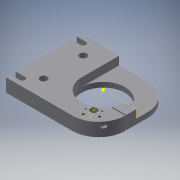
# Autodesk Inventor part: v2_tri_mount
Saved by Autodesk Inventor 2019 (Build 230136000, 136)
## iProperties
Created: 2017-03-10
Part Number: v2_tri_mount
Material: Generic
Document SubType Name: Modeling
Designer: richp
Density: 1 g/cm^3
Appearance: Default
mount_radius: 0.964 in
fov_diameter: 0.300 in
tri_angle: 120.00 deg
hole_diameter: 1.639 in
main_aperture_diameter: 1.639 in
Author: richp
Autodesk Inventor part; units mm, degrees
ref_plane "YZ Plane" through (0, 0, 0) normal (1, 0, 0) x (0, 1, 0)
ref_plane "XZ Plane" through (0, 0, 0) normal (0, 1, 0) x (-1, 0, 0)
ref_plane "XY Plane" through (0, 0, 0) normal (0, 0, 1) x (1, 0, 0)
sketch "Sketch1" plane through (0, 0, 0) normal (0, 1, 0) x (-1, 0, 0)
  line L0 (-54.2742, 0) -> (84.3226, 0) construction
  line L1 (-6.35, -36.068) -> (57.15, -36.068)
  line L2 (57.15, -36.068) -> (57.15, 36.068)
  line L3 (57.15, 36.068) -> (-6.35, 36.068)
  line L4 (-31.75, 10.668) -> (-31.75, -10.668)
  circle A0 centre (0, 0) radius 17 construction
  circle A1 centre (0, 0) radius 20.81
  line L5 (0, 0) -> (-18.9066, 32.7472) construction
  circle A2 centre (0, 0) radius 3.81 construction
  arc A3 (-6.35, 36.068) -> (-31.75, 10.668) centre (-6.35, 10.668) ccw
  arc A4 (-31.75, -10.668) -> (-6.35, -36.068) centre (-6.35, -10.668) ccw
  circle A5 centre (-12.2465, 21.2116) radius 1.6256 construction
  line L6 (0, 0) -> (31.1733, 53.9938) construction
  circle A6 centre (24.493, 0) radius 1.6256 construction
  circle A7 centre (-12.2465, -21.2116) radius 1.6256 construction
  circle A8 centre (-12.2465, 21.2116) radius 3.175 construction
  point P0 (-31.75, -36.068)
  point P1 (-31.75, 36.068)
  dimension "d0" = 72.136
  dimension "d1" = 88.9
  dimension "d2" = 34
  dimension "d3" = 3.81
  dimension "d4" = 31.75
  dimension "tri_angle" = 120
  dimension "fov_diameter" = 7.62
  dimension "d9" = 25.4
  dimension "d12" = 3.2512
  dimension "mount_radius" = 24.493
  dimension "d14" = 60
  dimension "d25" = 6.35
  dimension "main_aperture_diameter" = 41.62
  dimension "d67" = 2.0574
  dimension "d68" = 10.94
  constraints: 14 end point, 9 centre point, 6 point on line, 5 point on circle, 4 coincident, 4 tangent, 2 horizontal, 2 parallel, 2 symmetric about line, 1 equal radius, 1 perpendicular, 3 other
  measures "d0" distance of point (-31.75, 36.068) point (-31.75, -36.068)
  measures "d1" distance of L2.end point (-31.75, 36.068)
  measures "d2" diameter of A0
  measures "d3" radial gap between concentric circles of A1 A0
  measures "d4" distance from line of L5.start L4
  measures "tri_angle" angle of L0 L5
  measures "fov_diameter" diameter of A2
  measures "d9" radius of A3
  measures "d12" diameter of A5
  measures "mount_radius" distance of L5.start A5.centre
  measures "d14" angle of L0 L6
  measures "d25" diameter of A8
  measures "main_aperture_diameter" diameter of A1
  measures "d68" distance edge to line of A1 L4
extrude "Extrusion2" add sketch "Sketch1" against normal blind 12.7
sketch "Sketch12" plane through (0, 0, 0) normal (0, 1, 0) x (1, 0, 0)
  line L0 (0, 0) -> (18.9066, -32.7472) construction
  line L1 (12.2465, -21.2116) -> (8.7633, -23.2226) construction
  point P0 (7.2972, -24.0691)
  point P1 (17.1958, -18.3541)
  dimension "d94" = 11.43
  constraints: 2 end point, 1 perpendicular, 1 point on line, 1 symmetric about line
  measures "d94" distance of point (17.196, -18.354) point (7.297, -24.069)
sketch "Sketch13" plane through (0, 0, 0) normal (0, 1, 0) x (1, 0, 0)
  line L0 (0, 0) -> (18.9066, -32.7472) construction
  point P0 (12.2465, -21.2116)
hole "Hole4" at (12.2465, 0, 21.2116) direction (0, -1, 0) diameter 6.604 depth 25.4 tip angle 118
sketch "Sketch14" plane through (0, 0, 0) normal (0, 1, 0) x (1, 0, 0)
  line L0 (-112.042, 0) -> (81.9935, 0) projected
  line L1 (-58.42, 29.1592) -> (-48.26, 29.1592) construction
  line L2 (-58.42, 31.6484) -> (-48.26, 31.6484)
  line L3 (-48.26, 26.67) -> (-58.42, 26.67)
  arc A0 (-58.42, 31.6484) -> (-58.42, 26.67) centre (-58.42, 29.1592) ccw
  arc A1 (-48.26, 26.67) -> (-48.26, 31.6484) centre (-48.26, 29.1592) ccw
  line L4 (-58.42, -31.6484) -> (-48.26, -31.6484)
  line L5 (-48.26, -26.67) -> (-58.42, -26.67)
  arc A2 (-58.42, -26.67) -> (-58.42, -31.6484) centre (-58.42, -29.1592) ccw
  arc A3 (-48.26, -31.6484) -> (-48.26, -26.67) centre (-48.26, -29.1592) ccw
  point P0 (0, 0)
  point P1 (-53.34, 29.1592)
  dimension "d102" = 4.9784
  dimension "d103" = 48.26
  dimension "d104" = 29.1592
  dimension "d105" = 10.16
  constraints: 12 end point, 8 point on circle, 6 symmetric about line, 4 centre point, 4 tangent, 1 horizontal, 1 midpoint, 1 parallel, 2 other
  measures "d102" distance between parallel lines of L3 L2
  measures "d103" horizontal distance of point (0, 0) L3.start
  measures "d104" distance from line of L0 point (-53.34, 29.159)
  measures "d105" distance of L2.end L2.start
extrude "Extrusion11" cut sketch "Sketch14" against normal blind 25.4
sketch "Sketch16" plane through (0, 0, 0) normal (0, 1, 0) x (1, 0, 0)
  line L0 (-112.042, 0) -> (81.9935, 0) projected
  line L1 (0, 50.4952) -> (0, -50.4952) projected
  arc A0 (-20.81, 0) -> (-20.81, 0) centre (0, 0) ccw projected
  line L2 (-20.81, 81.7717) -> (-20.81, 0)
  line L3 (0, 0) -> (42.69, 0)
  line L4 (42.69, 0) -> (42.69, 81.7717)
  line L5 (42.69, 81.7717) -> (-20.81, 81.7717)
  line L6 (0, 0) -> (-20.81, 0)
  line L7 (-20.81, 0) -> (-37.279, 0)
  dimension "d112" = 63.5
  dimension "d113" = 81.7717
  dimension "d124" = 0
  constraints: 12 end point, 3 point on line, 2 vertical, 1 collinear, 1 perpendicular, 1 tangent, 2 other
  measures "d112" distance of L4.end L2.start
  measures "d113" distance of L3.end L4.end
  measures "d124" distance between parallel lines of L0 L3
extrude "Extrusion13" cut sketch "Sketch16" against normal blind 7.9375 contours A0 L1 L0 | L2 L5 L4 L0 A0 | L1 A0 L0 picked at (-13.6994, 1.5436) picked at (7.3346, 11.673)
sketch "Sketch17" plane through (0, -12.7, 0) normal (0, -1, 0) x (1, 0, 0)
  point P0 (0, 0)
  point P1 (7.2972, 24.0691)
  point P2 (17.1958, 18.3541)
hole "Hole6" at (7.2972, -12.7, 24.0691) at (17.1958, -12.7, 18.3541) direction (0, 1, 0) diameter 1.7018 depth 25.4 tip angle 118
sketch "Sketch18" plane through (0, 0, 0) normal (0, 1, 0) x (1, 0, 0)
  line L0 (0, 0) -> (18.9066, -32.7472) construction
  line L1 (7.2972, -24.0691) -> (11.5397, -31.4173) construction
  point P0 (17.1958, -18.3541)
  point P1 (10.4722, -29.5683)
  point P2 (20.3708, -23.8533)
  dimension "d125" = 6.35
  constraints: 2 end point, 1 parallel, 1 point on line, 1 symmetric about line
  measures "d125" distance of L1.start point (10.472, -29.568)
hole "Hole7" at (10.4722, 0, 29.5683) at (20.3708, 0, 23.8533) direction (0, -1, 0) diameter 2.159 depth 8.8646 tip angle 118
sketch "Sketch19" plane through (0, 0, 0) normal (0, 1, 0) x (1, 0, 0)
  line L0 (54.2742, 0) -> (-84.3226, 0) construction
  point P0 (0, 0)
  point P1 (0, 0)
  point P2 (-38.1, 19.05)
  point P3 (-38.1, -19.05)
  dimension "d133" = 38.1
  dimension "d134" = 38.1
  constraints: 1 symmetric about line
  measures "d133" horizontal distance of point (-38.1, 19.05) point (0, 0)
  measures "d134" distance of point (-38.1, -19.05) point (-38.1, 19.05)
hole "Hole8" at (-38.1, 0, 19.05) at (-38.1, 0, -19.05) direction (0, -1, 0) diameter 6.7564 depth 19.05 tip angle 118 clearance for "Flat Head Machine Screw (82)" size "1/4" standard "Ansi Unified Screw Threads"
sketch "Sketch20" plane through (0, 0, 0) normal (0, 1, 0) x (1, 0, 0)
  line L0 (31.75, -10.668) -> (15.3822, -10.668)
  line L1 (15.3822, -10.668) -> (15.3822, -9.652)
  line L2 (15.3822, -9.652) -> (31.75, -9.652)
  line L3 (31.75, -9.652) -> (31.75, -10.668)
  point P0 (0, 0)
  dimension "d142" = 1.016
  dimension "d143" = 16.3678
  constraints: 8 end point, 2 parallel, 1 horizontal, 1 perpendicular
  measures "d142" distance between parallel lines of L0 L2
  measures "d143" distance from line of L2.end L1
extrude "Extrusion14" cut sketch "Sketch20" against normal blind 25.4
sketch "Sketch21" plane through (31.75, 0, 0) normal (0, 0, -1) x (-1, 0, 0)
  line L0 (0, -7.9375) -> (0, 0) construction
  line L1 (0, -7.9375) -> (10.94, -7.9375) construction
  line L2 (10.94, 0) -> (10.94, -7.9375) construction
  line L3 (0, 0) -> (10.94, 0) construction
  line L4 (10.94, 0) -> (0, -7.9375) construction
  line L5 (0, 0) -> (25.4, 0) construction
  line L6 (0, -7.9375) -> (10.94, -7.9375) construction
  line L7 (0, 0) -> (10.94, -7.9375) construction
  point P0 (31.75, 0)
  point P1 (5.47, -3.9688)
  constraints: 4 end point, 1 midpoint
hole "Hole9" at (26.28, -3.9688, 0) direction (0, 0, 1) diameter 3.2766 depth 10.16 clearance for "Flat Head Machine Screw (82)" size "#4" standard "Ansi Unified Screw Threads"
sketch "Sketch22" plane through (31.75, 0, 10.668) normal (0, 0, -1) x (-1, 0, 0)
  point P0 (31.75, 0)
  point P1 (5.47, -3.9688)
hole "Hole10" at (26.28, -3.9688, 10.668) direction (0, 0, 1) diameter 3.302 depth 25.4 tip angle 118 thread size "8-32 UNC" class "2B" standard "ANSI Unified Screw Threads"
sketch "Sketch23" plane through (0, -12.7, 0) normal (0, -1, 0) x (1, 0, 0)
  line L0 (0, 0) -> (18.9066, 32.7472) construction
  arc A0 (17.8676, 10.668) -> (18.4362, 9.652) centre (0, 0) ccw projected
  arc A1 (31.75, 10.668) -> (6.35, 36.068) centre (6.35, 10.668) ccw projected
  circle A2 centre (13.5955, 23.5481) radius 6
  line L1 (6.5804, 20.67) -> (17.5284, 14.3493) construction
  circle A3 centre (12.2465, 21.2116) radius 3.302 construction
  dimension "d160" = 12
  constraints: 2 end point, 2 tangent, 1 centre point, 1 perpendicular, 1 point on line
  measures "d160" diameter of A2
extrude "Extrusion15" [suppressed]
equation "\"fov_diameter\" = 2 * d3"
equation "\"d14\" = 0.5 * tri_angle"
equation "\"d15\" = plate_thickness"
equation "\"plate_thickness\" = 12.7"
equation "\"magnet_depth\" = plate_thickness - pin_depth"
equation "\"hole_diameter\" = d2 + fov_diameter"
equation "\"pin_depth\" = 2.921"
body "Solid2"
